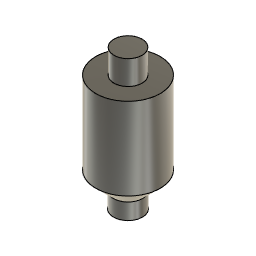
stud v2 (Autodesk Fusion 360 design; units mm, degrees)
Autodesk Fusion 360 part; units mm, degrees
sketch "Sketch1" plane through (0, 0, 0) normal (0, 0, 1) x (1, 0, 0)
  circle A0 centre (0, 0) radius 2
  dimension "d1" = 4
  constraint coincident A0.centre origin
  measures "d1" diameter of A0
extrude "Extrude1" add sketch "Sketch1" along normal blind 6.2
sketch "Sketch2" plane through (0, 0, 6.2) normal (0, 0, 1) x (-1, 0, 0)
  circle A0 centre (0, 0) radius 2
  circle A1 centre (0, 0) radius 0.875
  dimension "d4" = 1.75
  constraint coincident A0.centre A1.centre
  measures "d4" diameter of A1
extrude "Extrude2" add sketch "Sketch2" along normal blind 1.5 contours A1
chamfer "Chamfer2" distance 1.1 angle 45 1 edges at (-1.8647, -0.7232, 0)
extrude "Extrude4" add 1 faces at (0.4737, -0.323, 0) along direction (0, 0, -1) blind 1
